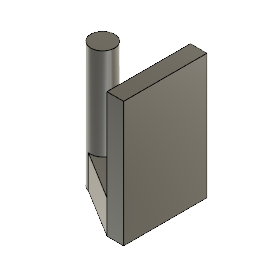
Desktrunk-Clip (Autodesk Fusion 360 design; units mm, degrees)
Autodesk Fusion 360 part; units mm, degrees
note: some values were not read from the file. Chosen so that the rebuilt part matches the saved one: which face or edge a step refers to; that a step has no effect; which pieces of a blend or face edit are solid.
sketch "Sketch1" plane through (0, 0, 0) normal (1, 0, 0) x (0, 1, 0)
  line L0 (-5, 6) -> (11.1286, 6)
  line L1 (11.1286, 6) -> (11.1286, -7.5034)
  line L2 (11.1286, -7.5034) -> (-5, -7.5034)
  line L3 (-5, -7.5034) -> (-5, 6)
  constraint horizontal L0
  constraint vertical L1
  constraint horizontal L2
  constraint vertical L3
sketch "Sketch2" plane through (0, 0, 0) normal (1, 0, 0) x (0, 1, 0)
  line L0 (-28, 22) -> (-16, 22)
  line L1 (-16, 22) -> (-16, 10.6443)
  line L2 (-16, 10.6443) -> (-36, 10.6443)
  line L3 (-36, 10.6443) -> (-28, 22)
  constraint horizontal L0
  constraint perpendicular L0 L1
  constraint perpendicular L1 L2
sketch "Sketch3" plane through (0, 0, 0) normal (0, 0, 1) x (1, 0, 0)
  circle A0 centre (-31.5, 17.5) radius 1.5811
sketch "Sketch4" plane through (0, 0, 0) normal (0, 0, 1) x (1, 0, 0)
  line L0 (-20, 25) -> (-5, 25)
  line L1 (-5, 25) -> (-5, 5)
  line L2 (-5, 5) -> (-20, 5)
  line L3 (-20, 5) -> (-20, 25)
  constraint horizontal L0
  constraint vertical L1
  constraint horizontal L2
  constraint vertical L3
sketch "Sketch5" plane through (0, 0, 2.8539) normal (0, 0, 1) x (-1, 0, 0)
  line L0 (20, -5) -> (5, -5)
  line L1 (5, -5) -> (5, -25)
  line L2 (5, -25) -> (20, -25)
  line L3 (20, -25) -> (20, -5)
  line L4 (13.5, -20) -> (10.5, -20)
  arc A0 (10.5, -18.5) -> (10.5, -20) centre (10.5, -19.25) ccw
  line L5 (10.5, -18.5) -> (13.5, -18.5)
  arc A1 (13.5, -20) -> (13.5, -18.5) centre (13.5, -19.25) ccw
  constraint horizontal L4
  constraint tangent L4 A0
  constraint tangent A0 L5
  constraint parallel L4 L5
  constraint tangent L5 A1
  constraint tangent L4 A1
sketch "Sketch6" plane through (0, 0, 2.8539) normal (0, 0, 1) x (-1, 0, 0)
  line L0 (13.5, -20) -> (10.5, -20)
  arc A0 (10.5, -18.5) -> (10.5, -20) centre (10.5, -19.25) ccw
  line L1 (10.5, -18.5) -> (13.5, -18.5)
  arc A1 (13.5, -20) -> (13.5, -18.5) centre (13.5, -19.25) ccw
  line L2 (20, -5) -> (5, -5)
  line L3 (5, -5) -> (5, -25)
  line L4 (5, -25) -> (20, -25)
  line L5 (20, -25) -> (20, -5)
  circle A2 centre (12, -7) radius 1
  dimension "d11" = 2
  measures "d11" diameter of A2
sketch "Sketch7" plane through (0, 0, 0) normal (0, 0, 1) x (1, 0, 0)
  line L0 (-5, 10) -> (-15, 10)
  line L1 (-15, 10) -> (-15, -32)
  line L2 (-15, -32) -> (-5, -32)
  line L3 (-5, -32) -> (-5, 10)
  dimension "d14" = 42
  dimension "d15" = 10
  constraint horizontal L0
  constraint vertical L1
  constraint horizontal L2
  constraint vertical L3
  measures "d14" distance of L0.start L2.end
  measures "d15" distance of L0.start L0.end
sketch "Sketch8" plane through (0, 0, 2) normal (0, 0, 1) x (-1, 0, 0)
  line L0 (5, 32) -> (5, -10)
  line L1 (5, -10) -> (15, -10)
  line L2 (15, -10) -> (15, 32)
  line L3 (15, 32) -> (5, 32)
  circle A0 centre (10, -6.5) radius 1.5
  dimension "d18" = 3
  measures "d18" diameter of A0
sketch "Sketch9" plane through (0, 0, 0) normal (0, 0, 1) x (1, 0, 0)
  line L0 (-15, -32) -> (-5, -32)
  line L1 (-15, 10) -> (-15, -32)
  line L2 (-12, -29) -> (-8, -29)
  line L3 (-8, -26) -> (-12, -26)
  ellipse E0 centre (-12, -27.5) end of major axis (-12, -29) minor radius 0.5003 (-12, -26) -> (-12, -29) ccw
  ellipse E1 centre (-8, -27.5) end of major axis (-8, -29) minor radius 0.5011 (-8, -29) -> (-8, -26) ccw
  constraint horizontal L2
sketch "Sketch10" plane through (0, 0, 0) normal (0, 0, 1) x (1, 0, 0)
  line L0 (-5, 10) -> (-15, 10)
  line L1 (15, -15) -> (35, -15)
  line L2 (15, -15) -> (15, -5)
  line L3 (15, -5) -> (35, -5)
  line L4 (35, -5) -> (35, -15)
  dimension "d27" = 20
  constraint parallel L0 L1
  constraint coincident L1 L2.start
  constraint perpendicular L1 L2
  constraint perpendicular L2 L3
  measures "d27" distance of L1.start L1.end
extrude "Extrude10" add sketch "Sketch10" along normal blind 1 makes body 1
sketch "Sketch11" plane through (0, 0, 0) normal (1, 0, 0) x (0, 1, 0)
  line L0 (-32, 0) -> (10, 0)
  line L1 (-5, 0) -> (-5, 1)
  line L2 (-15, 0) -> (-5, 0)
  line L3 (-5, 0) -> (-7.5, 3)
  line L4 (-7.5, 3) -> (-12.5, 3)
  line L5 (-12.5, 3) -> (-15, 0)
  point P0 (-15, 0)
  point P1 (-15, 0)
  constraint coincident P0 L2.start
  constraint coincident L0 L1.start
  constraint perpendicular L1 L2
  constraint coincident L1.start L2.end
  constraint perpendicular L1 L4
  constraint coincident P1 P0
extrude "Extrude11" add sketch "Sketch11" along normal blind 1 separate body makes body 2
move_body "Move3" bodies 2 to x (1, 0, 0) y (0, 1, 0) z (0, 0, 1) at (4, 0.7682, 0.6402)
sketch "Sketch12" plane through (0, 0, 0) normal (1, 0, 0) x (0, 1, 0)
  circle A0 centre (-2.5, 7.5) radius 1.25
  dimension "d32" = 2.5
  measures "d32" diameter of A0
extrude "Extrude12" add sketch "Sketch12" along normal blind 15 separate body makes body 3
move_face "MoveFace2" by (0, 0, 1) 1 faces at (4.3333, -8.3984, 3.6402) on bodies 2
move_body "Move4" bodies 2 to x (1, 0, 0) y (0, 1, 0) z (0, 0, 1) at (11, -0.3841, 0.3201)
move_body "Move5" bodies 1 to x (1, 0, 0) y (0, 1, 0) z (0, 0, 1) at (0, 0.4, 0)
sketch "Sketch13" plane through (15, 0, 0) normal (1, 0, 0) x (0, 1, 0)
move_face "MoveFace3" to x (1, 0, 0) y (0, 1, 0) z (0, 0, 1) at (20, 0, 0) 1 faces at (10, -1.2562, 7.3755) on bodies 3
move_body "Move6" bodies 3 to x (1, 0, 0) y (0, 1, 0) z (0, 0, 1) at (15, -7, -2)
sketch "Sketch14" plane through (16, 0, 0) normal (1, 0, 0) x (0, 1, 0)
sketch "Sketch15" plane through (0, 0, 0) normal (0, 0, 1) x (1, 0, 0)
  line L0 (15, -14.6) -> (35, -14.6)
  line L1 (30, -3.6592) -> (30, -16.2646)
  line L2 (30, -16.2646) -> (36, -16.2646)
  line L3 (36, -16.2646) -> (36, -3.5)
  line L4 (36, -3.5) -> (30, -3.6592)
  constraint perpendicular L0 L1
  constraint perpendicular L1 L2
  constraint perpendicular L2 L3
extrude "Extrude13" cut sketch "Sketch15" along normal blind 5 bodies 1
mesh "Mesh1" [no effect]
combine "Combine1" operation add target body 1 tool bodies 2 3
mesh "Mesh2" [no effect]
move_body "Move7" bodies 1 to x (0, 0, 1) y (0, 1, 0) z (-1, 0, 0) at (15, 0, -15)
mesh "Mesh3" [no effect]
move_face "OffsetFaces1" offset 1 1 faces at (15, -11.2667, 5) on bodies 1
extrude "Extrude14" add 3 faces at (15.3333, -7.9497, 0) (12.6799, -9.9531, 0) (14.0334, -14.6053, 0) along direction (0, 0, -1) blind 1.5 on bodies 1 bodies 1
sketch "Sketch17" plane through (0, 0, 0) normal (0, 1, 0) x (1, 0, 0)
cylinder "CylinderPrimitive2" add diameter 2.7 height 15 placed x (1, 0, 0) y (0, 1, 0) z (0, 0, 1) at (3, 4, 0) separate body makes body 4
box "BoxPrimitive1" add length 10 width 2 height 15 placed x (0, 1, 0) y (-1, 0, 0) z (0, 0, 1) at (11, 0, 0) separate body makes body 5
move_body "Move8" bodies 4 to x (1, 0, 0) y (0, 1, 0) z (0, 0, 1) at (0, 1, 0)
sketch "Sketch20" plane through (0, 0, 0) normal (0, 0, 1) x (1, 0, 0)
  line L0 (9, 0) -> (9, 10)
  line L1 (9, 10) -> (3.0071, 6.35)
  line L2 (3.0071, 6.35) -> (3, 3.7)
  line L3 (3, 3.7) -> (9, 0)
  circle A0 centre (3, 5) radius 1.35
  circle A1 centre (3, 5) radius 1.35
  constraint vertical L0
  constraint coincident L1.end A0
  constraint coincident L1.end A1
extrude "Extrude16" add sketch "Sketch20" along normal blind 3 contours L0 L1 L3 A0 A1 bodies 4 5
move_body "Move9" bodies 4 to x (1, 0, 0) y (0, 1, 0) z (0, 0, 1) at (5, 0, 0)
move_body "Move10" bodies 1 to x (1, 0, 0) y (0, 1, 0) z (0, 0, 1) at (-0.5, 0, 0)
move_face "MoveFace8" to x (1, 0, 0) y (0, 1, 0) z (0, 0, 1) at (2, 10, 0) 1 faces at (7.8029, 6.3355, 10) on bodies 4
move_face "MoveFace9" to x (1, 0, 0) y (0, 1, 0) z (0, 0, 1) at (0, 2, 0) 1 faces at (7.8029, 6.3355, 10) on bodies 4
cylinder "CylinderPrimitive3" add diameter 2.9 height 15 placed x (1, 0, 0) y (0, 1, 0) z (0, 0, 1) at (7.5, 10, 3) separate body makes body 6
move_body "Move11" bodies 6 to x (1, 0, 0) y (0, 1, 0) z (0, 0, 1) at (0.5, -5, 0)
extrude "Extrude17" cut 1 faces at (8.7175, 4.5745, 18) along direction (0, 0, -1) blind 3 on bodies 6 bodies 6
extrude "Extrude18" add 1 faces at (12.45, 5, 3) along direction (0, 0, 1) blind 1 on bodies 4 bodies 4 6
extrude "Extrude19" add 1 faces at (6.7229, 4.4747, 3) along direction (0, 0, -1) blind 3 on bodies 4 bodies 4
move_face "MoveFace10" to x (1, 0, 0) y (0, 1, 0) z (0, 0, 1) at (0.5, 0, 0) 1 faces at (7.9975, 6.45, 6.3333) on bodies 4
hidden bodies 1
